Autodesk Fusion 360 part; units mm, degrees
(part 2 of 2)
sketch "Sketch30" plane through (0, 0, 0) normal (0, -1, 0) x (1, 0, 0)
  line L0 (40, 0) -> (71.5, 0)
  line L1 (71.5, 0) -> (71.5, 10)
  line L2 (71.5, 10) -> (40, 10)
  line L3 (40, 10) -> (40, 0)
  line L4 (40, 10) -> (42, 10)
  line L5 (42, 10) -> (40, 0)
  line L6 (40, 0) -> (40, 10)
  line L7 (71.5, 10) -> (69.5, 10)
  line L8 (69.5, 10) -> (71.5, 0)
  line L9 (71.5, 0) -> (71.5, 10)
  dimension "d261" = 2
  constraint coincident L2.end L3.start
  constraint coincident L2 L4.end
  constraint coincident L0.start L3.end
  constraint coincident L1.end L2.start
  constraint perpendicular L1 L7
  constraint coincident L0.end L1.start
  measures "d261" distance of L1.end L7.end
sketch "Sketch31" plane through (71.5, 0, 0) normal (1, 0, 0) x (0, 0, -1)
  line L0 (0, 0) -> (0, 18)
  line L1 (0, 18) -> (-10, 18)
  line L2 (-10, 18) -> (-10, 0)
  line L3 (-10, 0) -> (0, 0)
  line L4 (-10, 0) -> (-10, 2)
  line L5 (-10, 2) -> (0, 0)
  line L6 (0, 0) -> (-10, 0)
  line L7 (-10, 18) -> (-10, 16)
  line L8 (-10, 16) -> (0, 18)
  line L9 (0, 18) -> (-10, 18)
  constraint coincident L2.end L3.start
  constraint coincident L2 L4.end
  constraint coincident L0.start L3.end
  constraint coincident L1.end L2.start
  constraint coincident L2 L7.end
  constraint coincident L0.end L1.start
extrude "Extrude32" cut sketch "Sketch31" against normal blind 40 contours L2 L3 L4 L5 L6 | L1 L2 L7 L8 L9 bodies 8
extrude "Extrude33" cut sketch "Sketch30" against normal blind 27 contours L2 L3 L4 L5 L6 | L1 L2 L7 L8 L9 bodies 8
shell "Shell9" thickness 1 removed faces 1 at (50.5, 12, 0) on bodies 8
sketch "Sketch32" plane through (0, 0, 9) normal (0, 0, -1) x (-1, 0, 0)
  line L0 (-68.6802, 15.1802) -> (-68.6802, 2.8198)
  line L1 (-68.6802, 2.8198) -> (-42.8198, 2.8198)
  line L2 (-42.8198, 2.8198) -> (-42.8198, 15.1802)
  line L3 (-42.8198, 15.1802) -> (-68.6802, 15.1802)
  line L4 (-56.3, 7) -> (-55.2, 7)
  line L5 (-55.2, 7) -> (-55.2, 11)
  line L6 (-55.2, 11) -> (-56.3, 11)
  line L7 (-56.3, 11) -> (-56.3, 7)
  line L8 (-53.75, 8.375) -> (-57.75, 8.375)
  line L9 (-57.75, 8.375) -> (-57.75, 9.625)
  line L10 (-57.75, 9.625) -> (-53.75, 9.625)
  line L11 (-53.75, 9.625) -> (-53.75, 8.375)
  line L12 (-57.3, 6) -> (-54.2, 6)
  line L13 (-54.2, 6) -> (-54.2, 12)
  line L14 (-54.2, 12) -> (-57.3, 12)
  line L15 (-57.3, 12) -> (-57.3, 6)
  line L16 (-58.75, 10.625) -> (-52.75, 10.625)
  line L17 (-52.75, 10.625) -> (-52.75, 7.375)
  line L18 (-52.75, 7.375) -> (-58.75, 7.375)
  line L19 (-58.75, 7.375) -> (-58.75, 10.625)
  dimension "d275" = 3.1
  dimension "d276" = 6
  dimension "d279" = 6
  dimension "d280" = 3.25
  constraint horizontal L4
  constraint vertical L5
  constraint horizontal L6
  constraint vertical L7
  constraint horizontal L8
  constraint vertical L9
  constraint horizontal L10
  constraint vertical L11
  constraint horizontal L12
  constraint vertical L13
  constraint horizontal L14
  constraint vertical L15
  constraint horizontal L16
  constraint vertical L17
  constraint horizontal L18
  constraint vertical L19
  measures "d275" distance of L12.start L12.end
  measures "d276" distance of L12.start L14.end
  measures "d279" distance of L16.start L16.end
  measures "d280" distance of L16.start L18.end
extrude "Extrude34" add sketch "Sketch32" along normal blind 9 contours L4 L5 L7 L12 L13 L15 L18 | L7 L8 L15 L18 | L5 L8 L13 L18 | L8 L9 L10 L15 L16 L18 L19 | L8 L10 L11 L13 L16 L17 L18 | L7 L10 L15 L16 | L5 L10 L13 L16 | L5 L6 L7 L13 L14 L15 L16 bodies 8
fillet "Fillet9" radius 1 8 edges at (55.75, 16, 10) (41, 17, 5) (42, 9, 10) (41, 1, 5) (55.75, 2, 10) (70.5, 17, 5) (69.5, 9, 10) (70.5, 1, 5) on bodies 8
move_body "Move13" bodies 8 to x (1, 0, 0) y (0, 1, 0) z (0, 0, 1) at (-55.7506, -8.335, 12.2427)
move_body "Move14" bodies 1 to x (1, 0, 0) y (0, 1, 0) z (0, 0, 1) at (70, 0, 0)
move_body "Move15" bodies 2 to x (1, 0, 0) y (0, 1, 0) z (0, 0, 1) at (-80, 0, 0)
move_body "Move16" bodies 3 to x (1, 0, 0) y (0, 1, 0) z (0, 0, 1) at (100, 0, 0)
move_body "Move17" bodies 4 to x (1, 0, 0) y (0, 1, 0) z (0, 0, 1) at (140, 0, 0)
move_body "Move18" bodies 5 to x (1, 0, 0) y (0, 1, 0) z (0, 0, 1) at (180, 0, 0)
move_body "Move19" bodies 6 to x (1, 0, 0) y (0, 1, 0) z (0, 0, 1) at (220, 0, 0)
move_body "Move20" bodies 7 to x (1, 0, 0) y (0, 1, 0) z (0, 0, 1) at (270, 0, 0)
move_body "Move21" bodies 8 to x (1, 0, 0) y (0, 1, 0) z (0, 0, 1) at (40, 0, 0)
move_body "Move22" bodies 2 to x (1, 0, 0) y (0, 1, 0) z (0, 0, 1) at (40, 0, 0)
equation "d31 = 18 mm + 18 mm + 18 mm + 18 mm + 18 mm + 18 mm"
equation "d70 = 18 mm + 4.5 mm"
equation "d100 = 18 mm + 18 mm"
equation "d150 = 18 mm + 9 mm"
equation "d174 = 18 mm + 18 mm + 4.5 mm"
equation "d212 = 18 mm + 18 mm + 9 mm + 4.5 mm"
equation "d257 = 18 mm + 9 mm + 4.5 mm"
